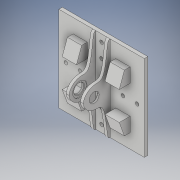
# Autodesk Inventor part: DoubleFork
Saved by Autodesk Inventor 2019 (Build 230136000, 136)
## iProperties
Created: 2018-06-02
Part Number: DoubleFork
Material: Generic
Document SubType Name: Modeling
Designer: Till
Density: 1 g/cm^3
Appearance: Default
Author: Till
Autodesk Inventor part; units mm, degrees
sketch "Sketch1" plane through (0, 0, 0) normal (0, 0, 1) x (1, 0, 0)
  line L0 (-60, 60) -> (60, 60)
  line L1 (60, 60) -> (60, -60)
  line L2 (60, -60) -> (-60, -60)
  line L3 (-60, -60) -> (-60, 60)
  line L4 (-84, 0) -> (84, 0) projected
  line L5 (0, -84) -> (0, 84) projected
  point P0 (0, 0)
  dimension "d0" = 120
  dimension "d1" = 120
  constraints: 8 end point, 2 parallel, 1 horizontal, 1 perpendicular, 2 other
  measures "d0" distance of L0.start L0.end
  measures "d1" distance of L0.end L1.end
extrude "Extrusion1" add sketch "Sketch1" along normal blind 5
ref_plane "Work Plane1" through (8, 0, 0) normal (1, 0, 0) x (0, 1, 0)
ref_plane "Work Plane2" through (-8, 0, 0) normal (1, 0, 0) x (0, 1, 0)
sketch "Sketch3" plane through (-8, 0, 0) normal (1, 0, 0) x (0, 1, 0)
  line L0 (-60, 0) -> (60, 0) projected
  line L1 (-60, 0) -> (-60, 5) projected
  line L2 (60, 5) -> (-60, 5) projected
  line L3 (60, 0) -> (60, 5) projected
  line L4 (0, -8.6187) -> (0, 51.7122) projected
  spline S0 degree 4 poles (0, 42.5) (8.8891, 42.5) (22.7497, 25.8839) (-1.7531, 12.5643) (56.3286, 8.8728) (60, 8.4213) (60, 5) knots 0 0 0 0 0 0.40951 0.65951 1 1 1 1 1
  line L5 (60, 0) -> (60, 5) projected
  spline S1 degree 4 poles (0, 42.5) (-8.8891, 42.5) (-22.7497, 25.8839) (1.7531, 12.5643) (-56.3286, 8.8728) (-60, 8.4213) (-60, 5) knots 0 0 0 0 0 0.40951 0.65951 1 1 1 1 1
  line L6 (-60, 0) -> (-60, 5) projected
  point P0 (0, 0)
  point P1 (15, 27.5)
  point P2 (18, 16.25)
  point P3 (56.7857, 8.2143)
  point P4 (0, 27.5)
  point P5 (-15, 27.5)
  point P6 (-18, 16.25)
  point P7 (-56.7857, 8.2143)
  dimension "d6" = 15
  dimension "d7" = 15
  dimension "d8" = 22.5
  dimension "d9" = 0
  dimension "d10" = 11.25
  dimension "d11" = 18
  dimension "d12" = 3.2143
  dimension "d13" = 3.2143
  constraints: 4 vertical, 3 symmetric about line, 2 point on line, 10 other
  measures "d6" distance from line of L4 point (15, 27.5)
  measures "d7" distance of point (0, 42.5) point (0, 27.5)
  measures "d8" distance from line of L2 point (0, 27.5)
  measures "d9" vertical distance of point (0, 27.5) point (15, 27.5)
  measures "d10" distance from line of point (18, 16.25) L2
  measures "d11" distance from line of L4 point (18, 16.25)
  measures "d12" distance from line of L2 point (56.786, 8.214)
  measures "d13" distance from line of point (56.786, 8.214) L3
extrude "Extrusion2" add sketch "Sketch3" against normal blind 4 contours S1 L4 L2 | L4 S0 L2
sketch "Sketch4" plane through (8, 0, 0) normal (1, 0, 0) x (0, 1, 0)
  spline S0 degree 4 poles (0, 42.5) (-8.8891, 42.5) (-22.7497, 25.8839) (1.7531, 12.5643) (-56.3286, 8.8728) (-60, 8.4213) (-60, 5) knots 0 0 0 0 0 0.40951 0.65951 1 1 1 1 1 projected
  spline S1 degree 4 poles (60, 5) (60, 8.4213) (56.3286, 8.8728) (-1.7531, 12.5643) (22.7497, 25.8839) (8.8891, 42.5) (0, 42.5) knots 0 0 0 0 0 0.34049 0.59049 1 1 1 1 1 projected
  line L0 (-60, 5) -> (60, 5) projected
  point P0 (0, 0)
  constraints: 2 other
extrude "Extrusion3" add sketch "Sketch4" along normal blind 4
sketch "Sketch7" plane through (-8, 0, 0) normal (1, 0, 0) x (0, 0, -1)
  line L0 (16.3435, 0) -> (-55.4779, 0) projected
  line L1 (-5, 60) -> (-5, -60) projected
  point P0 (0, 0)
  point P1 (-27.5, 0)
  point P2 (-42.5, 0)
  dimension "d35" = 0
  dimension "forkCurvature" = 15
  constraints: 1 point on line, 4 other
  measures "d35" distance from line of L0 point (-27.5, 0)
  measures "forkCurvature" distance of point (-27.5, 0) point (-42.5, 0)
hole "Hole3" at (-8, 0, 27.5) direction (-1, 0, 0) diameter 14 end through all both
sketch "Sketch8" plane through (-8, 0, 0) normal (1, 0, 0) x (0, 0, -1)
  circle A0 centre (-27.5, 0) radius 7 projected
  point P0 (0, 0)
  constraints: 1 coincident
hole "Hole4" at (-8, 0, 27.5) direction (-1, 0, 0) diameter 20.2 depth 1
fillet "Fillet1" radius 0.6 1 edges at (-9, 0, 34.5) inverted yes
sketch "Sketch9" plane through (8, 0, 0) normal (-1, 0, 0) x (0, 0, 1)
  circle A0 centre (27.5, 0) radius 7 projected
  point P0 (0, 0)
  constraints: 1 coincident
hole "Hole5" at (8, 0, 27.5) direction (1, 0, 0) diameter 20.2 depth 1
fillet "Fillet2" radius 0.6 1 edges at (9, 0, 34.5) inverted yes
sketch "Sketch10" plane through (0, 0, 5) normal (0, 0, 1) x (1, 0, 0)
  line L0 (0, -84) -> (0, 84) projected
  point P0 (0, 0)
  point P1 (0, 50)
  point P2 (0, 30)
  point P3 (-30, 0)
  point P4 (-50, 0)
  point P5 (0, -30)
  point P6 (0, -50)
  point P7 (30, 0)
  point P8 (50, 0)
  dimension "d60" = 30
  dimension "d61" = 50
  dimension "d64" = 360
  constraints: 2 point on line, 9 other
  measures "d60" distance of point (0, 0) point (0, 30)
  measures "d61" distance of point (0, 0) point (0, 50)
hole "Hole6" at (0, 50, 5) at (0, 30, 5) at (-30, 0, 5) at (-50, 0, 5) at (0, -30, 5) at (0, -50, 5) at (30, 0, 5) at (50, 0, 5) direction (0, 0, -1) diameter 5 end through all
ref_plane "Work Plane3" through (30, 0, 0) normal (1, 0, 0) x (0, 1, 0)
ref_plane "Work Plane4" through (-30, 0, 0) normal (1, 0, 0) x (0, 1, 0)
sketch "Sketch12" plane through (30, 0, 0) normal (1, 0, 0) x (0, 1, 0)
  line L0 (-60, 5) -> (60, 5) projected
  circle A0 centre (0, 27.5) radius 7 projected
  line L1 (-40, 5) -> (-40, 12.9412)
  line L2 (-20, 20.2206) -> (-20, 5)
  line L3 (-60, 5) -> (60, 5) projected
  line L4 (-40, 12.9412) -> (-20, 20.2206)
  line L5 (-20, 5) -> (-40, 5)
  line L6 (0, -8.5) -> (0, 51) projected
  line L7 (20, 5) -> (20, 20.2206)
  line L8 (40, 5) -> (40, 12.9412)
  line L9 (40, 12.9412) -> (20, 20.2206)
  line L10 (20, 5) -> (40, 5)
  line L11 (60, 5) -> (-60, 5) projected
  point P0 (0, 0)
  dimension "d75" = 20
  dimension "d76" = 40
  dimension "d77" = 20
  dimension "d78" = 40
  dimension "d84" = 20
  dimension "d85" = 20
  constraints: 16 end point, 6 point on line, 2 collinear, 2 parallel, 1 perpendicular, 1 vertical
  measures "d75" distance from line of A0.centre L2
  measures "d76" distance from line of A0.centre L1
  measures "d77" distance between parallel lines of L6 L7
  measures "d78" distance between parallel lines of L6 L8
  measures "d84" angle of L4 L0
  measures "d85" angle of L0 L9
extrude "Extrusion4" add sketch "Sketch12" along normal mid plane 20 contours L1 L4 L2 L0 | L7 L9 L8 L0
sketch "Sketch13" plane through (-30, 0, 0) normal (1, 0, 0) x (0, 1, 0)
  line L0 (-40, 5) -> (-20, 5) projected
  line L1 (-40, 5) -> (-40, 12.9412) projected
  line L2 (-40, 12.9412) -> (-20, 20.2206) projected
  line L3 (-20, 20.2206) -> (-20, 5) projected
  line L4 (40, 12.9412) -> (40, 5) projected
  line L5 (20, 5) -> (40, 5) projected
  line L6 (20, 5) -> (20, 20.2206) projected
  line L7 (20, 20.2206) -> (40, 12.9412) projected
  point P0 (0, 0)
extrude "Extrusion5" add sketch "Sketch13" along normal mid plane 20
equation "\"d1\" = d0"
equation "\"d6\" = forkCurvature"
equation "\"d7\" = forkCurvature"
equation "\"d8\" = 1.5 * d7"
equation "\"d10\" = 0.5 * d8"
equation "\"d11\" = 1.2 * d6"
equation "\"d12\" = 0.142857 * d8"
equation "\"d13\" = d12"
equation "\"d77\" = d75"
equation "\"d78\" = d76"
body "Solid1"
